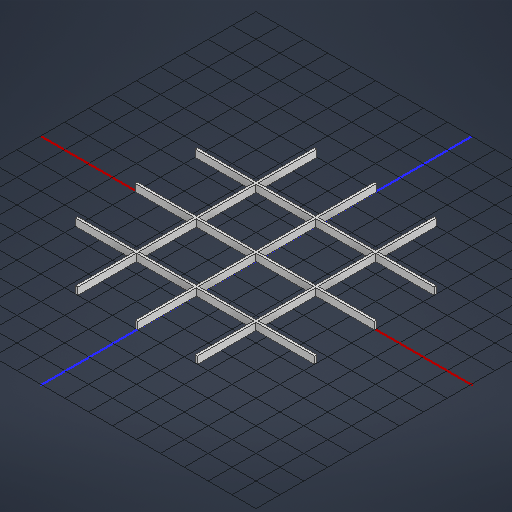
# Autodesk Inventor part: Square Holder Support
Saved by Autodesk Inventor 2026 (Build 300175000, 175)
## iProperties
Created: 2025-04-18
Part Number: Square Holder Support
Material: Generic
Document SubType Name: Modeling
Designer: ckyiu
Density: 1 g/cm^3
Appearance: Default
Author: ckyiu
Autodesk Inventor part; units mm, degrees
ref_plane "YZ Plane" through (0, 0, 0) normal (1, 0, 0) x (0, 1, 0)
ref_plane "XZ Plane" through (0, 0, 0) normal (0, 1, 0) x (-1, 0, 0)
ref_plane "XY Plane" through (0, 0, 0) normal (0, 0, 1) x (1, 0, 0)
sketch "Sketch1" plane through (0, 0, 0) normal (0, 1, 0) x (-1, 0, 0)
  line L0 (-100, 100) -> (100, 100) construction
  line L1 (100, 100) -> (100, -100) construction
  line L2 (100, -100) -> (-100, -100) construction
  line L3 (-100, -100) -> (-100, 100) construction
  line L4 (-100, 100) -> (100, -100) construction
  line L5 (100, 100) -> (-100, -100) construction
  line L6 (100, 0) -> (-100, 0) construction
  line L7 (0, 100) -> (0, -100) construction
  line L8 (0, 100) -> (100, 0) construction
  line L9 (100, 50) -> (-100, 50) construction
  line L10 (100, 0) -> (0, -100) construction
  line L11 (100, -50) -> (-100, -50) construction
  line L12 (50, 100) -> (50, -100) construction
  line L13 (-50, 100) -> (-50, -100) construction
  line L14 (0, 100) -> (-100, 0) construction
  line L15 (100, 51) -> (-100, 51)
  line L16 (-100, 51) -> (-100, 49)
  line L17 (-100, 49) -> (100, 49)
  line L18 (100, 49) -> (100, 51)
  line L19 (100, 1) -> (-100, 1)
  line L20 (-100, 1) -> (-100, -1)
  line L21 (-100, -1) -> (100, -1)
  line L22 (100, -1) -> (100, 1)
  line L23 (100, -49) -> (-100, -49)
  line L24 (-100, -49) -> (-100, -51)
  line L25 (-100, -51) -> (100, -51)
  line L26 (100, -51) -> (100, -49)
  line L27 (51, 100) -> (49, 100)
  line L28 (49, 100) -> (49, -100)
  line L29 (49, -100) -> (51, -100)
  line L30 (51, -100) -> (51, 100)
  line L31 (1, 100) -> (-1, 100)
  line L32 (-1, 100) -> (-1, -100)
  line L33 (-1, -100) -> (1, -100)
  line L34 (1, -100) -> (1, 100)
  line L35 (-49, 100) -> (-51, 100)
  line L36 (-51, 100) -> (-51, -100)
  line L37 (-51, -100) -> (-49, -100)
  line L38 (-49, -100) -> (-49, 100)
  point P0 (0, 0)
  point P1 (50, 50)
  point P2 (50, -50)
  point P3 (-50, 50)
  point P4 (51, 49)
  point P5 (51, 51)
  point P6 (49, 51)
  point P7 (1, 51)
  point P8 (-1, 51)
  point P9 (-49, 51)
  point P10 (-51, 51)
  point P11 (-51, 49)
  point P12 (-51, 1)
  point P13 (-51, -1)
  point P14 (-51, -49)
  point P15 (-51, -51)
  point P16 (-49, -51)
  point P17 (-1, -51)
  point P18 (1, -51)
  point P19 (49, -51)
  point P20 (51, -51)
  point P21 (51, -49)
  point P22 (51, -1)
  point P23 (51, 1)
  point P24 (49, -1)
  point P25 (49, -49)
  point P26 (1, -49)
  point P27 (1, -1)
  point P28 (-1, -49)
  point P29 (-49, -49)
  point P30 (-49, -1)
  point P31 (-1, -1)
  point P32 (-1, 1)
  point P33 (-49, 1)
  point P34 (-49, 49)
  point P35 (-1, 49)
  point P36 (49, 49)
  point P37 (49, 1)
  point P38 (1, 1)
  point P39 (1, 49)
  dimension "d0" = 200
  dimension "d1" = 200
  dimension "d3" = 1
  dimension "d4" = 1
  dimension "d5" = 1
  dimension "d6" = 1
  dimension "d7" = 1
  dimension "d8" = 1
  dimension "d9" = 1
  dimension "d10" = 1
  dimension "d11" = 1
  dimension "d12" = 1
  dimension "d13" = 1
  dimension "d14" = 1
  constraints: 78 end point, 24 point on line, 14 parallel, 11 perpendicular, 9 midpoint, 7 horizontal
  measures "d0" distance of L1.end L2.end
  measures "d1" distance of L0.end L1.end
  measures "d3" distance between parallel lines of L9 L15
  measures "d4" distance between parallel lines of L9 L17
  measures "d5" distance between parallel lines of L19 L6
  measures "d6" distance between parallel lines of L6 L21
  measures "d7" distance between parallel lines of L23 L11
  measures "d8" distance between parallel lines of L11 L25
  measures "d9" distance between parallel lines of L12 L30
  measures "d10" distance between parallel lines of L12 L28
  measures "d11" distance between parallel lines of L7 L34
  measures "d12" distance between parallel lines of L7 L32
  measures "d13" distance between parallel lines of L13 L38
  measures "d14" distance between parallel lines of L13 L36
extrude "Extrusion1" add sketch "Sketch1" along normal blind 6 contours L18 L17 L30 L15 | L30 L17 L28 L15 | L15 L28 L27 L30 | L28 L17 L34 L15 | L30 L19 L28 L17 | L34 L17 L32 L15 | L15 L32 L31 L34 | L30 L21 L28 L19 | L19 L22 L21 L30 | L32 L17 L38 L15 | L34 L19 L32 L17 | L28 L21 L34 L19 | L30 L23 L28 L21 | L38 L17 L36 L15 | L15 L36 L35 L38 | L34 L21 L32 L19 | L30 L25 L28 L23 | L23 L26 L25 L30 | L36 L17 L16 L15 | L38 L19 L36 L17 | L32 L21 L38 L19 | L34 L23 L32 L21 | L28 L25 L34 L23 | L30 L29 L28 L25 | L38 L21 L36 L19 | L34 L25 L32 L23 | L36 L21 L20 L19 | L38 L23 L36 L21 | L32 L25 L38 L23 | L34 L33 L32 L25 | L38 L25 L36 L23 | L36 L25 L24 L23 | L38 L37 L36 L25
equation "\"d0\" = chessboard_length"
equation "\"d1\" = chessboard_width"
equation "\"d3\" = 0.5 * square_holder_support_width"
equation "\"d4\" = d3"
equation "\"d5\" = d3"
equation "\"d6\" = d3"
equation "\"d7\" = d3"
equation "\"d8\" = d3"
equation "\"d9\" = d3"
equation "\"d10\" = d3"
equation "\"d11\" = d3"
equation "\"d12\" = d3"
equation "\"d13\" = d3"
equation "\"d14\" = d3"
equation "\"d15\" = square_holder_support_height"
equation "\"square_holder_support_width\" = 2"
equation "\"square_holder_support_height\" = 6"
equation "\"chessboard_length\" = 200"
equation "\"chessboard_width\" = 200"
body "Solid1"
